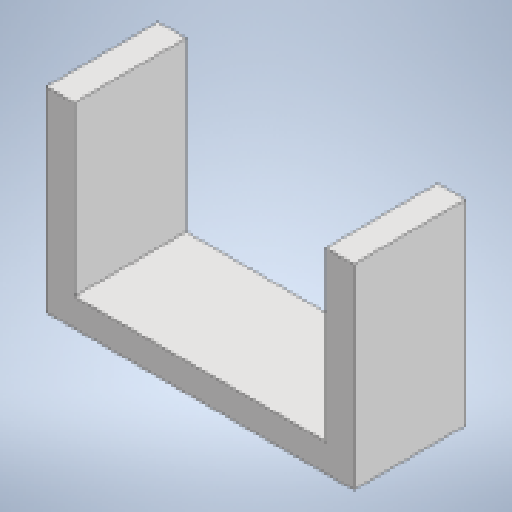
# Autodesk Inventor part: track z2101
Saved by Autodesk Inventor 2025.3 (Build 293356000, 356)
## iProperties
Created: 2026-04-19
Part Number: track z2101
Material: Generic
Document SubType Name: Modeling
Designer: kamal
Density: 1 g/cm^3
Appearance: Default
Author: kamal
Autodesk Inventor part; units mm, degrees
ref_plane "YZ Plane" through (0, 0, 0) normal (1, 0, 0) x (0, 1, 0)
ref_plane "XZ Plane" through (0, 0, 0) normal (0, 1, 0) x (-1, 0, 0)
ref_plane "XY Plane" through (0, 0, 0) normal (0, 0, 1) x (1, 0, 0)
sketch "Sketch1" plane through (0, 0, 0) normal (0, 0, 1) x (1, 0, 0)
  line L0 (22.5, 15) -> (-22.5, 15) construction
  line L1 (-22.5, 15) -> (-22.5, -15)
  line L2 (-22.5, -15) -> (22.5, -15)
  line L3 (22.5, -15) -> (22.5, 15)
  line L4 (22.5, 15) -> (-22.5, -15) construction
  line L5 (-22.5, 15) -> (22.5, -15) construction
  line L6 (-27.5, -20) -> (-27.5, 15)
  line L7 (-27.5, 20) -> (27.5, 20) construction
  line L8 (27.5, 20) -> (27.5, 15) construction
  line L9 (27.5, -20) -> (-27.5, -20)
  line L10 (-22.5, 15) -> (-27.5, 15)
  line L11 (22.5, 15) -> (27.5, 15)
  line L12 (-27.5, 15) -> (-27.5, 20) construction
  line L13 (27.5, 15) -> (27.5, -20)
  point P0 (0, 0)
  dimension "d0" = 45
  dimension "d1" = 30
  dimension "d2" = 5
  dimension "d3" = 5
  dimension "d4" = 5
  dimension "d5" = 40
  constraints: 28 end point, 7 parallel, 5 perpendicular, 2 midpoint, 1 horizontal, 1 point on line
  measures "d0" distance of L2.end L1.end
  measures "d1" distance of L1.end L0.end
  measures "d2" distance between parallel lines of L1 L6
  measures "d3" distance between parallel lines of L13 L3
  measures "d4" distance between parallel lines of L11 L7
  measures "d5" distance between parallel lines of L7 L9
extrude "Extrusion1" add sketch "Sketch1" along normal blind 7.126
body "Solid1"
